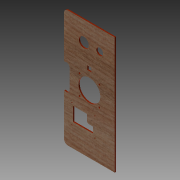
# Autodesk Inventor part: binnenplaat
Saved by Autodesk Inventor 2015 (Build 190159000, 159)
## iProperties
Created: 2015-12-31
Part Number: binnenplaat
Material: Generic
Document SubType Name: Modeling
Designer: david
Density: 1 g/cm^3
Appearance: White Oak - Natural Medium Gloss
Mass: 96.3167 g
Surface Area: 685.917 cm^2
Volume: 96.3167 cm^3
Author: david
Autodesk Inventor part; units mm, degrees
ref_plane "YZ Plane" through (0, 0, 0) normal (1, 0, 0) x (0, 1, 0)
ref_plane "XZ Plane" through (0, 0, 0) normal (0, 1, 0) x (-1, 0, 0)
ref_plane "XY Plane" through (0, 0, 0) normal (0, 0, 1) x (1, 0, 0)
sketch "Sketch1" plane through (0, 0, 0) normal (0, 1, 0) x (-1, 0, 0)
  line L0 (64, -147.5) -> (-64, -147.5)
  line L1 (-64, -147.5) -> (-64, 147.5)
  line L2 (-64, 147.5) -> (64, 147.5)
  line L3 (64, 147.5) -> (64, -147.5)
  line L4 (64, -147.5) -> (-64, 147.5) construction
  line L5 (-64, -147.5) -> (64, 147.5) construction
  point P0 (0, 0)
  dimension "d0" = 128
  dimension "d1" = 295
  constraints: 12 end point, 2 midpoint, 2 parallel, 1 horizontal, 1 perpendicular
  measures "d0" distance of L1.end L2.end
  measures "d1" distance of L0.end L1.end
extrude "Extrusion1" add sketch "Sketch1" along normal blind 3
sketch "Sketch2" plane through (0, 0, 0) normal (0, -1, 0) x (1, 0, 0)
  line L0 (-57.5, 25) -> (-57.5, -25) construction
  line L1 (-65, 25) -> (-65, -25)
  line L2 (-50, -25) -> (-50, 25)
  arc A0 (-50, 25) -> (-65, 25) centre (-57.5, 25) ccw
  arc A1 (-65, -25) -> (-50, -25) centre (-57.5, -25) ccw
  line L3 (-57.5, 0) -> (-7.5, 0) construction
  point P0 (0, 0)
  dimension "d4" = 25
  dimension "d5" = 90
  dimension "d6" = 15
  dimension "d7" = 50
  constraints: 10 end point, 4 point on circle, 4 tangent, 2 centre point, 1 horizontal, 1 midpoint, 1 parallel, 1 perpendicular, 1 vertical
  measures "d4" distance of L3.start L0.end
  measures "d5" angle of L0 L3
  measures "d6" diameter of A1
  measures "d7" distance from line of point (0, 0) L2
extrude "Extrusion2" cut sketch "Sketch2" against normal blind 3
sketch "Sketch3" plane through (0, 0, 0) normal (0, -1, 0) x (1, 0, 0)
  line L0 (30, -30) -> (-30, -30)
  line L1 (-30, -30) -> (-30, 30)
  line L2 (-30, 30) -> (30, 30)
  line L3 (30, 30) -> (30, -30)
  line L4 (30, -30) -> (-30, 30) construction
  line L5 (-30, -30) -> (30, 30) construction
  circle A0 centre (-25, -25) radius 2.2
  circle A1 centre (-25, 25) radius 2.2
  circle A2 centre (25, 25) radius 2.2
  circle A3 centre (25, -25) radius 2.2
  circle A4 centre (0, 0) radius 27.5
  dimension "d10" = 60
  dimension "d11" = 60
  dimension "d12" = 4.4
  dimension "d13" = 5
  dimension "d14" = 4.4
  dimension "d15" = 4.4
  dimension "d16" = 4.4
  dimension "d17" = 5
  dimension "d18" = 5
  dimension "d19" = 5
  dimension "d20" = 55
  constraints: 12 end point, 5 centre point, 4 midpoint, 4 point on line, 2 parallel, 1 horizontal, 1 perpendicular
  measures "d10" distance of L1.end L2.end
  measures "d11" distance of L0.end L1.end
  measures "d12" diameter of A0
  measures "d13" distance from line of L1 A0.centre
  measures "d14" diameter of A1
  measures "d15" diameter of A3
  measures "d16" diameter of A2
  measures "d17" distance from line of L1 A1.centre
  measures "d18" distance from line of L3 A2.centre
  measures "d19" distance from line of L3 A3.centre
  measures "d20" diameter of A4
extrude "Extrusion3" cut sketch "Sketch3" against normal blind 3 contours A0 | A1 | A2 | A3 | A4
sketch "Sketch5" plane through (0, 0, 0) normal (0, -1, 0) x (1, 0, 0)
  circle A0 centre (14, -97.5) radius 1.375
  circle A1 centre (-44, -97.5) radius 1.375
  circle A2 centre (-44, -48.5) radius 1.375
  circle A3 centre (14, -48.5) radius 1.375
  line L0 (-64, 147.5) -> (-64, -147.5) projected
  line L1 (-64, -147.5) -> (64, -147.5) projected
  point P0 (0, 0)
  dimension "d23" = 2.75
  dimension "d24" = 2.75
  dimension "d25" = 2.75
  dimension "d26" = 2.75
  dimension "d27" = 58
  dimension "d28" = 58
  dimension "d29" = 49
  dimension "d30" = 20
  dimension "d31" = 50
  dimension "d32" = 50
  dimension "d33" = 20
  dimension "d36" = 49
  constraints: 4 centre point
  measures "d23" diameter of A0
  measures "d24" diameter of A1
  measures "d25" diameter of A3
  measures "d26" diameter of A2
  measures "d27" distance of A0.centre A1.centre
  measures "d28" distance of A3.centre A2.centre
  measures "d29" distance of A3.centre A0.centre
  measures "d30" distance from line of L0 A1.centre
  measures "d31" distance from line of L1 A1.centre
  measures "d32" distance from line of L1 A0.centre
  measures "d33" distance from line of L0 A2.centre
  measures "d36" distance of A1.centre A2.centre
extrude "Extrusion4" cut sketch "Sketch5" against normal blind 3
sketch "Sketch6" plane through (0, 0, 0) normal (0, -1, 0) x (1, 0, 0)
  line L0 (-40, -89.5) -> (-6, -89.5)
  line L1 (-6, -69.5) -> (-6, -55.5)
  line L2 (-7, -54.5) -> (-40, -54.5)
  line L3 (-41, -55.5) -> (-41, -88.5)
  circle A0 centre (-44, -97.5) radius 1.375 projected
  circle A1 centre (-44, -48.5) radius 1.375 projected
  line L4 (-6, -89.5) -> (8, -89.5)
  line L5 (9, -88.5) -> (9, -75.5)
  line L6 (8, -74.5) -> (-1, -74.5)
  line L7 (-6, -74.5) -> (-6, -89.5)
  arc A2 (-6, -69.5) -> (-1, -74.5) centre (-1, -69.5) ccw
  arc A3 (9, -75.5) -> (8, -74.5) centre (8, -75.5) ccw
  arc A4 (8, -89.5) -> (9, -88.5) centre (8, -88.5) ccw
  arc A5 (-41, -88.5) -> (-40, -89.5) centre (-40, -88.5) ccw
  arc A6 (-40, -54.5) -> (-41, -55.5) centre (-40, -55.5) ccw
  arc A7 (-6, -55.5) -> (-7, -54.5) centre (-7, -55.5) ccw
  point P0 (0, 0)
  point P1 (9, -74.5)
  point P2 (9, -89.5)
  dimension "d39" = 3
  dimension "d43" = 6
  dimension "d58" = 15
  dimension "d59" = 15
  dimension "d60" = 5
  dimension "d61" = 1
  constraints: 16 end point, 12 point on circle, 12 tangent, 6 centre point, 6 point on line, 4 equal radius, 4 parallel, 2 horizontal, 2 perpendicular
  measures "d39" distance from line of A0.centre L3
  measures "d43" distance from line of L2 A1.centre
  measures "d58" distance of L7.start point (9, -74.5)
  measures "d59" distance of point (9, -74.5) point (9, -89.5)
  measures "d60" radius of A2
  measures "d61" radius of A3
extrude "Extrusion5" cut sketch "Sketch6" against normal blind 3 contours A5 L3 A6 L2 A7 L1 A2 L6 A3 L5 A4 L4 L0
sketch "Sketch8" plane through (0, 0, 0) normal (0, -1, 0) x (1, 0, 0)
  circle A0 centre (-14, 97.5) radius 12.5
  line L0 (64, 147.5) -> (-64, 147.5) projected
  line L1 (-64, 147.5) -> (-64, 28.7417) projected
  circle A1 centre (26, 97.5) radius 8.5
  point P0 (0, 0)
  dimension "d44" = 25
  dimension "d45" = 50
  dimension "d46" = 50
  dimension "d49" = 17
  dimension "d50" = 50
  dimension "d51" = 40
  constraints: 2 centre point
  measures "d44" diameter of A0
  measures "d45" distance from line of L0 A0.centre
  measures "d46" distance from line of L1 A0.centre
  measures "d49" diameter of A1
  measures "d50" distance from line of L0 A1.centre
  measures "d51" distance of A0.centre A1.centre
extrude "Extrusion6" cut sketch "Sketch8" against normal blind 3
fillet "Fillet1" radius 2 2 edges at (-64, 1.5, 28.7417) (-64, 1.5, -28.7417)
sketch "Sketch9" plane through (0, 0, 0) normal (0, -1, 0) x (1, 0, 0)
  line L0 (-5, 51.815) -> (5, 51.815)
  line L1 (5, 51.815) -> (5, 41.815)
  line L2 (5, 41.815) -> (-5, 41.815)
  line L3 (-5, 41.815) -> (-5, 51.815)
  line L4 (-5, 51.815) -> (5, 41.815) construction
  line L5 (5, 51.815) -> (-5, 41.815) construction
  point P0 (0, 0)
  point P1 (0, 46.815)
  dimension "d53" = 10
  dimension "d54" = 10
  dimension "d55" = 0
  constraints: 12 end point, 2 midpoint, 2 parallel, 1 horizontal, 1 perpendicular
  measures "d53" distance of L1.end L2.end
  measures "d54" distance of L0.end L1.end
  measures "d55" horizontal distance of point (0, 46.815) point (0, 0)
extrude "Extrusion7" cut sketch "Sketch9" against normal blind 10
fillet "Fillet2" radius 10 2 edges at (-64, 1.5, 147.5) (-64, 1.5, -147.5)
body "Solid1"
